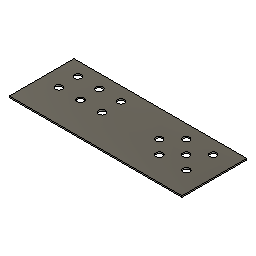
pb oanel v2 (Autodesk Fusion 360 archive; units mm, degrees)
design "pb oanel"
Autodesk Fusion 360 part; units mm, degrees
sketch "Sketch1" plane through (0, 0, 0) normal (0, 0, 1) x (1, 0, 0)
  line L0 (203.2, 76.2) -> (-203.2, 76.2)
  line L1 (-203.2, 76.2) -> (-203.2, -76.2)
  line L2 (-203.2, -76.2) -> (203.2, -76.2)
  line L3 (203.2, -76.2) -> (203.2, 76.2)
  line L4 (203.2, 76.2) -> (-203.2, -76.2) construction
  line L5 (-203.2, 76.2) -> (203.2, -76.2) construction
  dimension "d1" = 406.4
  dimension "d2" = 152.4
  constraint horizontal L0
  constraint perpendicular L0 L1
  constraint parallel L0 L2
  constraint parallel L1 L3
  constraint coincident L4 origin
  constraint coincident L5 origin
  measures "d1" distance of L1.end L2.end
  measures "d2" distance of L0.end L1.end
extrude "Extrude1" add sketch "Sketch1" along normal blind 3.175
sketch "Sketch2" plane through (0, 0, 3.175) normal (0, 0, 1) x (-1, 0, 0)
  line L0 (-203.2, 76.2) -> (-203.2, -76.2)
  line L1 (-203.2, -76.2) -> (203.2, -76.2)
  line L2 (203.2, -76.2) -> (203.2, 76.2)
  line L3 (203.2, 76.2) -> (-203.2, 76.2)
  circle A0 centre (162.56, -44.45) radius 7.9375
  circle A1 centre (60.96, -44.45) radius 7.9375
  line L4 (203.2, -44.45) -> (-203.2, -44.45) construction
  line L5 (203.2, -60.325) -> (-203.2, -60.325) construction
  circle A2 centre (162.56, -44.45) radius 10.795 construction
  line L6 (172.6056, -60.325) -> (-27.8584, -60.325) construction
  line L7 (-27.8584, -60.325) -> (-27.8584, -69.85) construction
  line L8 (-27.8584, -69.85) -> (172.6056, -69.85) construction
  line L9 (172.6056, -69.85) -> (172.6056, -60.325) construction
  circle A3 centre (162.56, 0) radius 7.9375
  circle A4 centre (111.76, 0) radius 7.9375
  circle A5 centre (60.96, 0) radius 7.9375
  line L10 (203.2, 0) -> (-203.2, 0) construction
  line L11 (203.2, -15.875) -> (-203.2, -15.875) construction
  line L12 (183.6475, -15.875) -> (19.338, -15.875) construction
  line L13 (19.338, -15.875) -> (19.338, -25.4) construction
  line L14 (19.338, -25.4) -> (183.6475, -25.4) construction
  line L15 (183.6475, -25.4) -> (183.6475, -15.875) construction
  circle A6 centre (111.76, -44.45) radius 7.9375
  dimension "button" = 15.875
  dimension "d7" = 15.875
  dimension "d12" = 15.875
  dimension "d13" = 21.59
  dimension "d14" = 9.525
  dimension "d17" = 9.525
  dimension "d22" = 15.875
  dimension "d23" = 15.875
  dimension "d24" = 15.875
  dimension "d25" = 50.8
  dimension "d26" = 50.8
  dimension "d28" = 44.45
  dimension "d29" = 15.875
  dimension "d85" = 60.96
  dimension "d86" = 60.96
  dimension "d88" = 152.4
  dimension "d89" = 406.4
  dimension "d96" = 10.0456
  dimension "d105" = 9.525
  dimension "d106" = 9.525
  dimension "d128" = 101.6
  dimension "d129" = 15.875
  dimension "d130" = 50.8
  constraint coincident L2 L4.start
  constraint coincident L0 L4.end
  constraint perpendicular L0 L4
  constraint coincident A0.centre L4
  constraint coincident A1.centre L4
  constraint coincident L2 L5.start
  constraint coincident L0 L5.end
  constraint perpendicular L0 L5
  constraint concentric A0 A2
  constraint coincident L5
  constraint coincident L2 L10.start
  constraint coincident L0 L10.end
  constraint perpendicular L0 L10
  constraint coincident A3.centre L10
  constraint coincident A4.centre L10
  constraint coincident A5.centre L10
  constraint coincident L2 L11.start
  constraint coincident L0 L11.end
  constraint perpendicular L0 L11
  constraint horizontal origin A5.centre
  constraint coincident L11
  constraint coincident L4 A6.centre
  measures "button" diameter of A0
  measures "d7" diameter of A1
  measures "d12" distance of L4 L5
  measures "d13" diameter of A2
  measures "d17" distance of L5 L8
  measures "d22" diameter of A3
  measures "d23" diameter of A4
  measures "d24" diameter of A5
  measures "d25" distance of A3.centre A4.centre
  measures "d26" distance of A4.centre A5.centre
  measures "d28" distance of L4 L10
  measures "d29" distance of L10 L11
  measures "d85" horizontal distance of origin A1.centre
  measures "d86" distance of origin A5.centre
  measures "d88" distance of L0.start L0.end
  measures "d89" distance of L0.end L1.end
  measures "d96" distance of A0.centre L9
  measures "d106" distance of L11 L14
  measures "d128" distance of A1.centre A0.centre
  measures "d129" diameter of A6
  measures "d130" distance of A1.centre A6.centre
extrude "Extrude3" cut sketch "Sketch2" against normal blind 50.8 contours A0 | A1 | A3 | A4 | A5 | A6
sketch "Sketch3" plane through (0, 0, 3.175) normal (0, 0, 1) x (-1, 0, 0)
  circle A0 centre (111.76, 0) radius 7.9375
  circle A1 centre (162.56, -44.45) radius 7.9375
  circle A2 centre (60.96, 0) radius 7.9375
  circle A3 centre (162.56, 0) radius 7.9375
  circle A4 centre (60.96, -44.45) radius 7.9375
  line L0 (-203.2, 76.2) -> (-203.2, -76.2)
  line L1 (-203.2, -76.2) -> (203.2, -76.2)
  line L2 (203.2, -76.2) -> (203.2, 76.2)
  line L3 (203.2, 76.2) -> (-203.2, 76.2)
  circle A5 centre (-92.71, -44.45) radius 7.9375
  circle A6 centre (-92.71, 19.05) radius 7.9375
  circle A7 centre (-60.96, -12.7) radius 7.9375
  circle A8 centre (-124.46, -12.7) radius 7.9375
  line L4 (-92.71, -44.45) -> (-92.71, 19.05) construction
  line L5 (-60.96, -12.7) -> (-124.46, -12.7) construction
  line L6 (-72.6401, -60.325) -> (-119.2488, -60.325) construction
  line L7 (-87.0646, -60.325) -> (-106.5413, -60.325) construction
  line L8 (-106.5413, -60.325) -> (-106.5413, -69.85) construction
  line L9 (-106.5413, -69.85) -> (-87.0646, -69.85) construction
  line L10 (-87.0646, -69.85) -> (-87.0646, -60.325) construction
  line L11 (-84.0964, 3.175) -> (-85.2577, 3.175)
  line L12 (-85.2577, 3.175) -> (-106.3727, 3.175) construction
  line L13 (-86.9218, 3.175) -> (-101.4306, 3.175) construction
  line L14 (-101.4306, 3.175) -> (-101.4306, -6.35) construction
  line L15 (-101.4306, -6.35) -> (-86.9218, -6.35) construction
  line L16 (-86.9218, -6.35) -> (-86.9218, 3.175) construction
  line L17 (-50.0842, -28.575) -> (-73.0383, -28.575) construction
  line L18 (-55.7529, -28.575) -> (-69.6326, -28.575) construction
  line L19 (-69.6326, -28.575) -> (-69.6326, -38.1) construction
  line L20 (-69.6326, -38.1) -> (-55.7529, -38.1) construction
  line L21 (-55.7529, -38.1) -> (-55.7529, -28.575) construction
  line L22 (-117.6854, -28.575) -> (-146.3556, -28.575) construction
  line L23 (-119.2474, -28.575) -> (-139.2811, -28.575) construction
  line L24 (-139.2811, -28.575) -> (-139.2811, -38.1) construction
  line L25 (-139.2811, -38.1) -> (-119.2474, -38.1) construction
  line L26 (-119.2474, -38.1) -> (-119.2474, -28.575) construction
  line L27 (-156.21, -44.45) -> (-156.21, 19.05) construction
  circle A9 centre (-156.21, -44.45) radius 7.9375
  circle A10 centre (-156.21, 19.05) radius 7.9375
  line L28 (-162.1579, 3.175) -> (-182.2496, 3.175) construction
  line L29 (-156.3761, -60.325) -> (-181.7712, -60.325) construction
  line L30 (-151.6704, -60.325) -> (-180.3361, -60.325) construction
  line L31 (-180.3361, -60.325) -> (-180.3361, -69.85) construction
  line L32 (-180.3361, -69.85) -> (-151.6704, -69.85) construction
  line L33 (-151.6704, -69.85) -> (-151.6704, -60.325) construction
  line L34 (-151.7847, 3.175) -> (-164.1052, 3.175) construction
  line L35 (-164.1052, 3.175) -> (-164.1052, -6.35) construction
  line L36 (-164.1052, -6.35) -> (-151.7847, -6.35) construction
  line L37 (-151.7847, -6.35) -> (-151.7847, 3.175) construction
  circle A11 centre (60.96, 0) radius 7.9375
  line L38 (-92.71, -44.45) -> (-92.71, -63.514) construction
  circle A12 centre (111.76, -44.45) radius 7.9375
  point P0 (-92.71, -12.7)
  point P1 (-156.21, -12.7)
  dimension "d6" = 15.875
  dimension "d11" = 25.4
  dimension "d46" = 15.875
  dimension "d47" = 15.875
  dimension "d48" = 15.875
  dimension "d49" = 15.875
  dimension "d51" = 63.5
  dimension "d52" = 63.5
  dimension "d56" = 15.875
  dimension "d57" = 9.525
  dimension "d58" = 9.525
  dimension "d59" = 15.875
  dimension "d60" = 9.525
  dimension "d61" = 9.525
  dimension "d62" = 15.875
  dimension "d63" = 9.525
  dimension "d64" = 9.525
  dimension "d65" = 15.875
  dimension "d66" = 9.525
  dimension "d67" = 9.525
  dimension "d71" = 15.875
  dimension "d72" = 15.875
  dimension "d73" = 9.525
  dimension "d74" = 9.525
  dimension "d75" = 15.875
  dimension "d76" = 15.875
  dimension "d77" = 9.525
  dimension "d78" = 9.525
  dimension "d82" = 38.1
  dimension "d98" = 63.5
  dimension "d99" = 63.5
  dimension "d100" = 31.75
  dimension "d101" = 31.75
  dimension "d102" = 31.75
  dimension "d103" = 31.75
  dimension "d104" = 406.4
  dimension "d109" = 60.96
  dimension "d110" = 63.5
  constraint coincident A5.centre L4.start
  constraint coincident A6.centre L4.end
  constraint vertical L4
  constraint coincident A7.centre L5.start
  constraint coincident A8.centre L5.end
  constraint horizontal L5
  constraint coincident L5 P0
  constraint coincident L4 P0
  constraint parallel L1 L6
  constraint coincident L6
  constraint perpendicular L4 L11
  constraint perpendicular L4 L12
  constraint coincident L12
  constraint horizontal L17
  constraint coincident L17
  constraint horizontal L22
  constraint coincident L22
  constraint parallel L4 L27
  constraint midpoint L27 P1
  constraint coincident L27.start A9.centre
  constraint coincident L27.end A10.centre
  constraint horizontal L28
  constraint horizontal L29
  constraint coincident L29
  constraint coincident L28
  constraint horizontal P0 P1
  constraint parallel L4 L38
  measures "d46" diameter of A5
  measures "d47" diameter of A6
  measures "d48" diameter of A7
  measures "d49" diameter of A8
  measures "d52" distance of L1 P0
  measures "d56" distance of A5.centre L6
  measures "d58" distance of L6 L9
  measures "d59" distance of A6.centre L12
  measures "d61" distance of L12 L15
  measures "d62" distance of A7.centre L17
  measures "d64" distance of L17 L20
  measures "d65" distance of A8.centre L22
  measures "d67" distance of L22 L25
  measures "d71" diameter of A9
  measures "d72" diameter of A10
  measures "d74" distance of L29 L32
  measures "d75" distance of L27.start L29
  measures "d76" distance of L27.end L28
  measures "d78" distance of L28 L36
  measures "d98" distance of A7.centre A8.centre
  measures "d99" distance of A5.centre A6.centre
  measures "d100" distance of A7.centre L4
  measures "d101" distance of A5.centre P0
  measures "d102" distance of P1 L27.start
  measures "d103" distance of A8.centre L27
  measures "d104" distance of L0.end L1.end
  measures "d109" horizontal distance of origin A7.centre
extrude "Extrude4" cut sketch "Sketch3" against normal blind 27.94 contours A5 | A6 | A7 | A8 | A9 | A10
sketch "Sketch4" plane through (0, 0, 3.175) normal (0, 0, 1) x (-1, 0, 0)
equation "d7 = d6"
equation "d22 = d6"
equation "d23 = d6"
equation "d24 = d6"
equation "d26 = d25"
equation "d46 = d6"
equation "d47 = d6"
equation "d48 = d6"
equation "d49 = d6"
equation "d61 = d78"
equation "d64 = d78"
equation "d71 = d6"
equation "d72 = d6"
equation "d85 = d89 * 0.15"
equation "d86 = d85"
equation "d99 = d98"
equation "d100 = d98 / 2"
equation "d101 = d100"
equation "d102 = d100"
equation "d103 = d100"
equation "d109 = d104 * 0.15"
equation "d110 = d98"
equation "d128 = d26 * 2"
equation "d129 = d7"
equation "d130 = d26"
equation "d111 = d101 + 0.25 in"
equation "d112 = d47"
equation "d113 = d47"
equation "d115 = d62"
equation "d117 = d115"
equation "d120 = d110 / 2"
equation "d121 = d113"
equation "d122 = d113"
equation "d123 = d110"
equation "d124 = d99"
